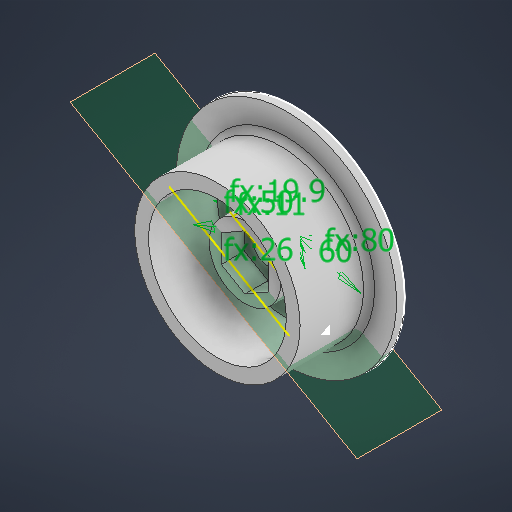
# Autodesk Inventor part: test_wheel_v1
Saved by Autodesk Inventor 2027.1 (Build 311270010, 270A)
## iProperties
Created: 2026-09-04
Part Number: test_wheel_v1
Material: Generic
Document SubType Name: Modeling
Designer: ajrcr
Density: 1 g/cm^3
Appearance: Default
Author: ajrcr
Autodesk Inventor part; units mm, degrees
ref_plane "YZ Plane" through (0, 0, 0) normal (1, 0, 0) x (0, 1, 0)
ref_plane "XZ Plane" through (0, 0, 0) normal (0, 1, 0) x (-1, 0, 0)
ref_plane "XY Plane" through (0, 0, 0) normal (0, 0, 1) x (1, 0, 0)
sketch "Sketch1" plane through (0, 0, 0) normal (0, 0, 1) x (1, 0, 0)
  circle A0 centre (0, 0) radius 30
  circle A1 centre (0, 0) radius 40
  circle A2 centre (0, 0) radius 25
  circle A3 centre (0, 0) radius 13
  circle A4 centre (0, 0) radius 5.5
  circle A5 centre (0, 0) radius 9.95 construction
  line L0 (0, 9.95) -> (8.617, 4.975)
  line L1 (8.617, 4.975) -> (8.617, -4.975)
  line L2 (8.617, -4.975) -> (0, -9.95)
  line L3 (0, -9.95) -> (-8.617, -4.975)
  line L4 (-8.617, -4.975) -> (-8.617, 4.975)
  line L5 (-8.617, 4.975) -> (0, 9.95)
  line L6 (0, 9.95) -> (0, -9.95) construction
  dimension "bolt_head_hub_WAC" = 19.9
  dimension "wheel_diam" = 60
  dimension "d1" = 80
  dimension "d4" = 50
  dimension "d5" = 26
  dimension "hub_id" = 11
  constraints: 14 end point, 7 coincident, 5 centre point, 1 vertical, 1 vertical alignment, 15 other
  measures "wheel_diam" diameter of A0
  measures "d1" diameter of A1
  measures "d4" diameter of A2
  measures "d5" diameter of A3
  measures "hub_id" diameter of A4
extrude "Extrusion1" add sketch "Sketch1" along normal blind 3 contours A0 | A1 | A2 | A3 | A4 | L0 L1 L2 L3 L4 L5
extrude "Extrusion2" add sketch "Sketch1" along normal blind 28 contours A0
extrude "Extrusion3" add sketch "Sketch1" along normal blind 18 contours A3 | L0 L1 L2 L3 L4 L5
extrude "Extrusion4" cut sketch "Sketch1" against normal blind 8.4 from surface at 18 contours L0 L1 L2 L3 L4 L5
extrude "Extrusion5" cut sketch "Sketch1" along normal up to surface (3 mm away) contours A4
fillet "Fillet1" radius 2 1 edges at (-30, 0, 3)
ref_plane "Work Plane1" through (-8.617, 4.975, 0) normal (-0.5, -0.8660254, 0) x (0, 0, -1)
equation "\"bolt_head_hub_WAC\" = bolt_WAC + 2 * printer_tolerance"
equation "\"d1\" = wheel_diam + 2 * flange_extra"
equation "\"d4\" = wheel_diam - 2 * wheel_thick"
equation "\"d5\" = bolt_head_hub_WAC + 2 * bolt_head_hub_clearance"
equation "\"hub_id\" = bolt_od + 2 * printer_tolerance"
equation "\"d8\" = track_w + flange_w"
equation "\"d10\" = flange_w + hub_height"
equation "\"track_w\" = 25"
equation "\"wheel_thick\" = 5"
equation "\"bolt_head_hub_clearance\" = 3.05"
equation "\"hub_height\" = 15"
equation "\"bolt_head_thick\" = 6.4"
equation "\"bolt_WAC\" = 18.9"
equation "\"printer_tolerance\" = 0.5"
equation "\"flange_extra\" = 10"
equation "\"bolt_od\" = 10"
equation "\"flange_w\" = 3"
body "Solid1"
